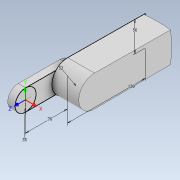
# Autodesk Inventor part: shank_inventor
Saved by Autodesk Inventor 2020 (Build 240168000, 168)
## iProperties
Created: 2021-01-07
Part Number: shank_inventor
Material: Generic
Document SubType Name: Modeling
Designer: DELL
Density: 1 g/cm^3
Appearance: Default
Author: DELL
Autodesk Inventor part; units mm, degrees
ref_plane "YZ Plane" through (0, 0, 0) normal (1, 0, 0) x (0, 1, 0)
ref_plane "XY Plane" through (0, 0, 0) normal (0, 0, 1) x (1, 0, 0)
ref_plane "UCS1: YZ Plane" through (0, 0, 0) normal (1, 0, 0) x (0, 1, 0)
sketch "Sketch2" plane through (0, 0, 0) normal (1, 0, 0) x (0, 1, 0)
  circle A0 centre (0, -70) radius 26
  line L0 (25, -200) -> (-25, -200)
  line L1 (0, -70) -> (0, -200) construction
  line L2 (-25.9992, -70.2001) -> (-25, -200)
  line L3 (25.9992, -70.2001) -> (25, -200)
  circle A1 centre (0, 0) radius 17.5
  circle A2 centre (0, -70) radius 17.5
  line L4 (17.5, 0) -> (17.5, -70)
  line L5 (-17.5, 0) -> (-17.5, -70)
  dimension "d1" = 52
  dimension "d3" = 50
  dimension "d25" = 130
  dimension "d26" = 35
  dimension "d27" = 70
  constraints: 12 end point, 6 point on circle, 4 tangent, 3 centre point, 2 coincident, 1 equal radius, 1 horizontal, 1 midpoint, 1 perpendicular, 1 vertical, 1 vertical alignment, 1 other
  measures "d1" diameter of A0
  measures "d3" distance of L0.start L0.end
  measures "d25" distance from line of L0 L1.start
  measures "d26" diameter of A1
  measures "d27" distance of L5.start L5.end
extrude "Extrusion1" add sketch "Sketch2" along normal blind 45 contours A0 L5 A2 L4 | A0 L4 A2 L5 | A2
extrude "Extrusion2" add sketch "Sketch2" against normal blind 45 from surface at 45 contours A0 L3 L0 L2
sketch "Sketch5" plane through (45, -25, -200) normal (0, 0, -1) x (-1, 0, 0)
  circle A0 centre (22.5, 25) radius 10
  line L0 (45, 50) -> (0, 50) projected
  line L1 (45, 50) -> (45, 0) projected
  point P0 (45, 25)
  point P1 (22.5, 50)
  point P2 (45, 25)
  dimension "d22" = 20
  constraints: 2 midpoint, 1 centre point, 1 horizontal alignment, 1 vertical alignment
  measures "d22" diameter of A0
extrude "Extrusion4" cut sketch "Sketch5" against normal blind 60
ref_plane "Work Plane1" through (22.5, 0, -70) normal (-1, 0, 0) x (0, 0, -1)
sketch "Sketch4" plane through (22.5, 0, -70) normal (-1, 0, 0) x (0, 0, -1)
  line L0 (130, -25) -> (130, 25) projected
  arc A0 (125.9592, -40) -> (130, 0) centre (-70, 0) ccw
  line L1 (125.9592, -40) -> (130, -40)
  line L2 (130, -40) -> (130, 0)
  line L3 (-115.2, 0) -> (201.2, 0) projected
  line L4 (-70, 0) -> (130, 0)
  point P0 (156, -25)
  point P1 (156, 25)
  point P2 (156, -25)
  dimension "d18" = 40
  constraints: 6 end point, 2 horizontal, 2 point on circle, 1 centre point, 1 coincident, 1 perpendicular, 2 other
  measures "d18" distance between parallel lines of L3 L1
revolve "Revolution1" cut sketch "Sketch4" angle 360 about axis through (22.5, 0, 0) along (0, 0, -1)
extrude "Extrusion5" add sketch "Sketch2" against normal blind 12 contours L5 A1 L4 A0 | A0 L4 A2 L5 | A1 | A2 picked at (-13.2429, -51.1519)
body "Solid1"
